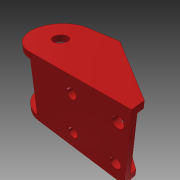
# Autodesk Inventor part: x_axis_cable_mount_a
Saved by Autodesk Inventor 2014 (Build 180170000, 170)
## iProperties
Created: 2013-12-04
Part Number: x_axis_cable_mount_a
Material: ABS Plastic
Document SubType Name: Modeling
Designer: buben
Density: 1.06 g/cm^3
Appearance: Light Red
Author: buben
Autodesk Inventor part; units mm, degrees
ref_plane "YZ Plane" through (0, 0, 0) normal (1, 0, 0) x (0, 1, 0)
ref_plane "XZ Plane" through (0, 0, 0) normal (0, 1, 0) x (-1, 0, 0)
sketch "Sketch1" plane through (0, 0, 0) normal (0, 0, 1) x (1, 0, 0)
  circle A0 centre (0, 0) radius 2.5
  arc A1 (0, 10) -> (0, -10) centre (0, 0) ccw
  line L0 (0, 10) -> (12, 10)
  line L1 (0, -10) -> (12, -10)
  line L2 (12, -10) -> (12, 10)
  dimension "d0" = 5
  dimension "d1" = 20
  dimension "d2" = 12
  constraints: 6 end point, 2 centre point, 2 coincident, 2 point on circle, 2 tangent, 1 horizontal, 1 parallel, 1 perpendicular
  measures "d0" diameter of A0
  measures "d1" diameter of A1
  measures "d2" distance from line of L2 point (0, 0)
extrude "Extrusion1" add sketch "Sketch1" along normal blind 2
sketch "Sketch5" plane through (0, 0, 0) normal (0, 0, -1) x (-1, 0, 0)
  circle A0 centre (0, 0) radius 2.5 projected
  line L0 (-12, -10) -> (0, -10)
  line L1 (0, -10) -> (0, -8)
  line L2 (0, -8) -> (-12, -8)
  line L3 (-12, -8) -> (-12, -10)
  line L4 (-12, 10) -> (-1, 10)
  line L5 (-1, 10) -> (-1, 8)
  line L6 (-1, 8) -> (-12, 8)
  line L7 (-12, 8) -> (-12, 10)
  dimension "d21" = 2
  dimension "d22" = 2
  dimension "d24" = 1
  constraints: 16 end point, 4 parallel, 2 horizontal, 2 perpendicular, 1 vertical alignment
  measures "d21" distance of L4.end L5.end
  measures "d22" distance of L0.end L1.end
  measures "d24" distance from line of A0.centre L5
extrude "Extrusion5" add sketch "Sketch5" along normal blind 2 contours L3 L2 L1 L0 | L4 L5 L6 L7
sketch "Sketch6" plane through (0, 0, -2) normal (0, 0, -1) x (-1, 0, 0)
  line L0 (-12, 8) -> (-1, 8) projected
  line L1 (-1, 8) -> (-1, 10) projected
  line L2 (-1, 9.162) -> (-2.5994, 8)
  line L3 (-2.5994, 8) -> (6.8052, -4.9443) construction
  line L4 (6.8052, -4.9443) -> (8.4046, -3.7823) construction
  line L5 (8.4046, -3.7823) -> (-1, 9.162) construction
  line L6 (-2.5994, 8) -> (-1, 8)
  line L7 (-1, 9.162) -> (-1, 8)
  point P0 (0, 0)
  dimension "d27" = 16
  dimension "d28" = 8
  dimension "d29" = 36
  constraints: 12 end point, 2 collinear, 2 perpendicular, 2 point on line, 1 parallel
  measures "d27" distance of L4.end L2.start
  measures "d28" distance from line of point (0, 0) L4
  measures "d29" angle of L0 L2
extrude "Extrusion6" cut sketch "Sketch6" against normal blind 2
ref_plane "Work Plane1" through (0, 0, -9) normal (0, 0, -1) x (-1, 0, 0)
mirror "Mirror1" about plane through (0, 0, -9) normal (0, 0, -1)
sketch "Sketch7" plane through (0, -10, -16) normal (0, 0, 1) x (1, 0, 0)
  line L0 (12, 0) -> (0, 0) projected
  line L1 (12, 2) -> (12, 0) projected
  line L2 (0, 2) -> (12, 2) projected
  line L3 (0, 0) -> (0, 2) projected
  line L4 (2.5994, 18) -> (1, 19.162) projected
  line L5 (12, 18) -> (2.5994, 18) projected
  line L6 (12, 20) -> (12, 18) projected
  line L7 (1, 20) -> (12, 20) projected
  line L8 (1, 19.162) -> (1, 20) projected
  point P0 (0, 10)
extrude "Extrusion7" add sketch "Sketch7" along normal blind 14
sketch "Sketch8" plane through (12, -10, 2) normal (1, 0, 0) x (0, 0, -1)
  line L0 (22, 20) -> (0, 20) projected
  line L1 (0, 0) -> (0, 20) projected
  line L2 (22, 0) -> (0, 0) projected
  line L3 (22, 0) -> (22, 20) projected
  line L4 (2, 18) -> (20, 18) projected
  line L5 (20, 2) -> (20, 18) projected
  line L6 (2, 2) -> (20, 2) projected
  line L7 (2, 2) -> (2, 18) projected
  point P0 (2, 10)
extrude "Extrusion8" add sketch "Sketch8" along normal blind 20
sketch "Sketch9" plane through (0, 0, -20) normal (0, 0, -1) x (-1, 0, 0)
  line L0 (-32, 10) -> (0, 10) projected
  line L1 (-32, -10) -> (-32, 10) projected
  line L2 (-32, -6) -> (-12, 10)
  dimension "d37" = 20
  dimension "d38" = 4
  constraints: 2 end point, 2 point on line
  measures "d37" distance of L0.start L2.end
  measures "d38" distance of L1.start L2.start
extrude "Extrusion9" cut sketch "Sketch9" against normal blind 22
sketch "Sketch10" plane through (0, -8, 0) normal (0, 1, 0) x (1, 0, 0)
  line L0 (32, 0) -> (0, 0) projected
  line L1 (32, 18) -> (32, 0) projected
  line L2 (0, 18) -> (32, 18) projected
  line L3 (15, 15) -> (29, 15) construction
  line L4 (29, 15) -> (29, 3) construction
  line L5 (29, 3) -> (15, 3) construction
  line L6 (15, 3) -> (15, 15) construction
  circle A0 centre (15, 3) radius 1.6
  circle A1 centre (29, 3) radius 1.6
  circle A2 centre (29, 15) radius 1.6
  circle A3 centre (15, 15) radius 1.6
  dimension "d41" = 3.2
  dimension "d42" = 3
  dimension "d43" = 3
  dimension "d44" = 3
  dimension "d45" = 14
  constraints: 8 end point, 4 centre point, 4 coincident, 3 equal radius, 2 parallel, 1 horizontal, 1 perpendicular
  measures "d41" diameter of A0
  measures "d42" distance between parallel lines of L1 L4
  measures "d43" distance between parallel lines of L2 L3
  measures "d44" distance between parallel lines of L0 L5
  measures "d45" distance between parallel lines of L4 L6
extrude "Extrusion10" cut sketch "Sketch10" against normal through all
body "Solid1"
